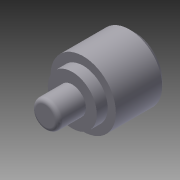
# Autodesk Inventor part: MU_Motor_Coupling_3
Saved by Autodesk Inventor 2011 SP2 (Build 150309200, 309)
## iProperties
Created: 2011-02-25
Part Number: MU_Motor_Coupling_3
Document SubType Name: Modeling
Designer: sungwook
Density: 2.71 g/cm^3
Material: Aluminum-6061-AHC
Mass: 0.0389141 g
Surface Area: 0.563916 cm^2
Volume: 0.0143594 cm^3
Author: sungwook
Autodesk Inventor part; units mm, degrees
ref_plane "YZ Plane" through (0, 0, 0) normal (1, 0, 0) x (0, 1, 0)
ref_plane "XZ Plane" through (0, 0, 0) normal (0, 1, 0) x (-1, 0, 0)
ref_plane "XY Plane" through (0, 0, 0) normal (0, 0, 1) x (1, 0, 0)
sketch "Sketch1" plane through (0, 0, 0) normal (0, 0, 1) x (1, 0, 0)
  circle A0 centre (0, 0) radius 1.2
  dimension "d0" = 2.4
  constraints: 1 centre point, 1 coincident
  measures "d0" diameter of A0
extrude "Extrusion1" add sketch "Sketch1" along normal blind 3.3
sketch "Sketch2" plane through (0, 0, 0) normal (0, 0, -1) x (-1, 0, 0)
  circle A0 centre (0, 0) radius 1.2 projected
  circle A1 centre (0, 0) radius 0.515
  dimension "d3" = 1.03
  constraints: 1 centre point, 1 coincident
  measures "d3" diameter of A1
sketch "Sketch4" plane through (0, 0, 3.3) normal (0, 0, 1) x (1, 0, 0)
  circle A0 centre (0, 0) radius 1.2 projected
  circle A1 centre (0, 0) radius 0.5
  circle A2 centre (0, 0) radius 1
  circle A3 centre (0, 0) radius 1.3
  dimension "d9" = 1
  dimension "d10" = 2
  dimension "d11" = 2.6
  constraints: 3 centre point, 3 coincident
  measures "d9" diameter of A1
  measures "d10" diameter of A2
  measures "d11" diameter of A3
extrude "Extrusion4" cut sketch "Sketch4" against normal blind 1.4 contours A0 | A2
sketch "Sketch5" plane through (0, 0, 1.9) normal (0, 0, 1) x (1, 0, 0)
  circle A0 centre (0, 0) radius 0.5 projected
  circle A1 centre (0, 0) radius 0.5 projected
  circle A2 centre (0, 0) radius 0.5 projected
  circle A3 centre (0, 0) radius 1.2 projected
  circle A4 centre (0, 0) radius 0.65
  circle A5 centre (0, 0) radius 0.3
  dimension "d14" = 1
  dimension "d15" = 1.3
  constraints: 2 centre point, 2 coincident
  measures "d14" diameter of A0
  measures "d15" diameter of A4
extrude "Extrusion5" [suppressed]
hole "Hole1" at (0, 0, 0) direction (0, 0, 1) diameter 1.05 depth 1.7 countersink diameter 1.5 countersink angle 90
sketch "Sketch6" plane through (0, 0, 1.9) normal (0, 0, 1) x (1, 0, 0)
  circle A0 centre (0, 0) radius 0.5 projected
  circle A1 centre (0, 0) radius 1.2 projected
  circle A2 centre (0, 0) radius 0.9
  dimension "d25" = 1.8
  constraints: 1 centre point, 1 coincident
  measures "d25" diameter of A2
extrude "Extrusion6" add sketch "Sketch6" along normal blind 0.4 contours A2
fillet "Fillet1" radius 0.15 1 edges at (-0.5, 0, 3.3)
fillet "Fillet2" [suppressed]
chamfer "Chamfer1" distance 0.2 angle 45 1 edges at (-1.2, 0, 0)
body "Solid1"
